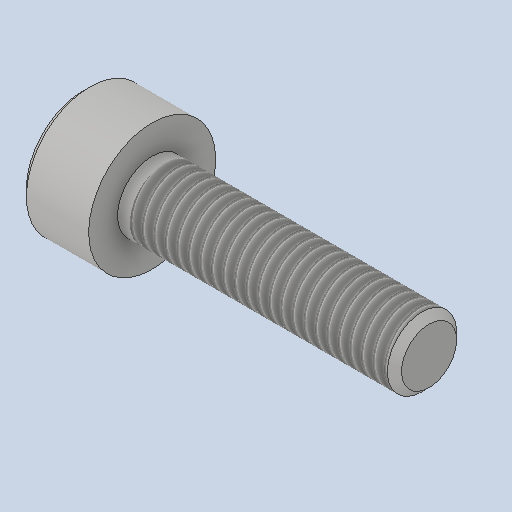
# Autodesk Inventor part: SNSX-M3-12-88
Saved by Autodesk Inventor 2025.1 (Build 291241020, 241B)
## iProperties
Created: 2024-11-07
Part Number: SNSX-M3-12-88
Material: Generic
Catalog Web Link: www.cadenas.de
Description: SNSX-88-High Intensity Socket Head Cap Screw
Vendor: NBK
Document SubType Name: Modeling
Designer: psAdmin
Manufacturer: NBK
Mass: 0.145193 g
Surface Area: 2.23071 cm^2
Volume: 0.145193 cm^3
Density: 1 g/cm^3
Appearance: PSOLRGB-175-175-175
Category: PARTsolutions
Company: NBK
PSOL_IDENT_0: {$CADENAS_DATA/23d-libs/nbk/e_nedzi_com/screws_made_with_sp_mat/snsx_88.prj},167 {VTYP=3D},{NB=SNSX-
PSOL_IDENT_1: M3-12-88},{LINA=SNSX-M3-12-88},{NN=SNSX-88},{DATE=05.11.2024 03:11:07},{GEOMDATE=09.12.2014 07:20:35
PSOL_IDENT_2: },{VERSION=},{LINEID=40},{WBVAR=},{WBNUMERIC=}  {NB=SNSX-M3-12-88},{LINA=SNSX-M3-12-88},{KT=DUMMY},{
PSOL_IDENT_3: CN=SNSX-M3-12-88},{SS=8.8},{M=M3},{L=12},{D1=5.5},{L1=3},{B=2.5},{L2=all thread},{MASS=1.10},{NDM=3}
PSOL_IDENT_4: ,{KDM=2.387},{LX=12}
NB: SNSX-M3-12-88
NN: SNSX-88
NT: High Intensity Socket Head Cap Screw
NBSYN: $CN.
LINA: SNSX-M3-12-88
CATALOG: NBK (Nabeya Bi-tech Kaisha
CN: SNSX-M3-12-88
SS: 8.8
M: M3
L: 12
D1: 5.5
L1: 3
B: 2.5
L2: Full Thread
MASS: 1.1
SUPPLIER: NBK
ARTICLENO: SNSX-M3-12-88
BOMINFO: SNSX-M3-12-88
CREATOR: CADENAS GmbH
Title: SNSX-M3-12-88
Author: Cadenas PARTsolutions
Comments: High Intensity Socket Head Cap Screw
Autodesk Inventor part; units mm, degrees
ref_plane "YZ Plane" through (0, 0, 0) normal (1, 0, 0) x (0, 1, 0)
ref_plane "XZ Plane" through (0, 0, 0) normal (0, 1, 0) x (-1, 0, 0)
ref_plane "XY Plane" through (0, 0, 0) normal (0, 0, 1) x (1, 0, 0)
sketch "Sketch_1" plane through (0, 0, 0) normal (0, 0, 1) x (1, 0, 0)
  line L0 (12, 0) -> (-3, 0)
  line L1 (-3, 0) -> (-3, 2.45)
  line L2 (-3, 2.45) -> (-2.7, 2.75)
  line L3 (-2.7, 2.75) -> (0, 2.75)
  line L4 (0, 2.75) -> (0, 1.5)
  line L5 (0, 1.5) -> (11.6935, 1.5)
  line L6 (11.6935, 1.5) -> (12, 1.1935)
  line L7 (12, 1.1935) -> (12, 0)
  line L8 (12, 0) -> (-3, 0)
  constraints: 18 end point
revolve "Revolution1" add sketch "Sketch_1" angle 360 about axis through (12, 0, 0) along (1, 0, 0)
thread "Thread1" size "M3x0.5" class "6g" standard "ISO Metric profile" length 11.4691 offset 0.5309
sketch "Sketch_2" plane through (-3, 0, 0) normal (1, 0, 0) x (0, 0, -1)
  line L0 (-1.25, -0.7217) -> (0, -1.4434)
  line L1 (0, -1.4434) -> (1.25, -0.7217)
  line L2 (1.25, -0.7217) -> (1.25, 0.7217)
  line L3 (1.25, 0.7217) -> (0, 1.4434)
  line L4 (0, 1.4434) -> (-1.25, 0.7217)
  line L5 (-1.25, 0.7217) -> (-1.25, -0.7217)
  constraints: 12 end point
extrude "Extrusion1" cut sketch "Sketch_2" along normal blind 1.8
body "Solid1"
